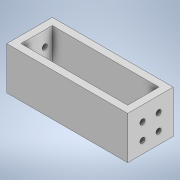
# Autodesk Inventor part: sidebracket
Saved by Autodesk Inventor 2020.1 (Build 241239000, 239)
## iProperties
Created: 2019-12-09
Part Number: sidebracket
Material: Generic
Document SubType Name: Modeling
Designer: tbloo
Density: 1 g/cm^3
Appearance: Default
Author: tbloo
Autodesk Inventor part; units mm, degrees
ref_plane "YZ Plane" through (0, 0, 0) normal (1, 0, 0) x (0, 1, 0)
ref_plane "XZ Plane" through (0, 0, 0) normal (0, 1, 0) x (-1, 0, 0)
ref_plane "XY Plane" through (0, 0, 0) normal (0, 0, 1) x (1, 0, 0)
sketch "Sketch1" plane through (0, 0, 0) normal (1, 0, 0) x (0, 1, 0)
  line L0 (0, 0) -> (30, 0)
  line L1 (30, 0) -> (30, 32)
  line L2 (30, 32) -> (0, 32)
  line L3 (0, 32) -> (0, 0)
  dimension "d0" = 30
  dimension "d1" = 32
  constraints: 8 end point, 2 parallel, 1 horizontal, 1 perpendicular
  measures "d0" distance of L2.end L1.end
  measures "d1" distance of L1.end L0.end
extrude "Extrusion1" add sketch "Sketch1" along normal blind 85
sketch "Sketch2" plane through (0, 30, 32) normal (0, 1, 0) x (1, 0, 0)
  line L0 (0, 32) -> (0, 0) projected
  line L1 (0, 0) -> (85, 0) projected
  line L2 (85, 32) -> (85, 0) projected
  line L3 (0, 32) -> (85, 32) projected
  line L4 (5, 5) -> (80, 5)
  line L5 (80, 5) -> (80, 27)
  line L6 (80, 27) -> (5, 27)
  line L7 (5, 27) -> (5, 5)
  line L8 (5, 5) -> (80, 27) construction
  line L9 (80, 5) -> (5, 27) construction
  point P0 (42.5, 16)
  dimension "d12" = 75
  dimension "d13" = 22
  constraints: 12 end point, 2 midpoint, 2 parallel, 1 horizontal, 1 perpendicular
  measures "d12" distance of L6.end L5.end
  measures "d13" distance of L5.end L4.end
extrude "Extrusion2" cut sketch "Sketch2" against normal blind 28 contours L7 L6 L5 L4
sketch "Sketch3" plane through (0, 0, 0) normal (-1, 0, 0) x (0, 0, 1)
  circle A0 centre (21.6569, 19.6569) radius 1.85
  circle A1 centre (21.6569, 8.3431) radius 1.85
  circle A2 centre (10.3431, 8.3431) radius 1.85
  circle A3 centre (10.3431, 19.6569) radius 1.85
  point P0 (0, 0)
  constraints: 4 centre point, 8 other
extrude "Extrusion3" cut sketch "Sketch3" against normal through all
body "Solid1"
